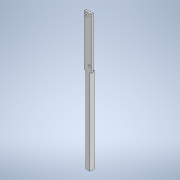
# Autodesk Inventor part: ArmV2
Saved by Autodesk Inventor 2021 (Build 250183000, 183)
## iProperties
Created: 2024-05-08
Part Number: ArmV2
Material: Generic
Document SubType Name: Modeling
Designer: brybr
Density: 1 g/cm^3
Appearance: Default
Author: brybr
Autodesk Inventor part; units mm, degrees
ref_plane "YZ Plane" through (0, 0, 0) normal (1, 0, 0) x (0, 1, 0)
ref_plane "XZ Plane" through (0, 0, 0) normal (0, 1, 0) x (-1, 0, 0)
ref_plane "XY Plane" through (0, 0, 0) normal (0, 0, 1) x (1, 0, 0)
sketch "Sketch1" plane through (0, 0, 0) normal (0, 0, 1) x (1, 0, 0)
  line L0 (-4, -30) -> (4, -30)
  line L1 (4, -30) -> (4, 30)
  line L2 (4, 30) -> (-4, 30)
  line L3 (-4, 30) -> (-4, -30)
  line L4 (-4, -30) -> (4, 30) construction
  line L5 (4, -30) -> (-4, 30) construction
  circle A0 centre (-2, 28) radius 1
  circle A1 centre (2, 28) radius 1
  circle A2 centre (-2, 25) radius 1
  circle A3 centre (2, -24) radius 1
  circle A4 centre (2, -23) radius 1
  point P0 (0, 0)
  point P1 (2.866, -23.5)
  point P2 (1.134, -23.5)
  dimension "d11" = 2
  dimension "d0" = 8
  dimension "d1" = 60
  dimension "d2" = 2
  dimension "d3" = 2
  dimension "d4" = 2
  dimension "d5" = 2
  dimension "d6" = 2
  dimension "d7" = 2
  dimension "d8" = 2
  dimension "d9" = 2
  dimension "d10" = 3
  dimension "d12" = 6
  dimension "d13" = 2
  dimension "d14" = 2
  constraints: 12 end point, 3 centre point, 2 midpoint, 2 parallel, 1 horizontal, 1 perpendicular, 6 other
  measures "d0" distance of L2.end L1.end
  measures "d1" distance of L1.end L0.end
  measures "d2" diameter of A0
  measures "d3" distance from line of L3 A0.centre
  measures "d4" distance from line of L2 A0.centre
  measures "d5" diameter of A1
  measures "d6" distance from line of L1 A1.centre
  measures "d7" distance from line of L2 A1.centre
  measures "d8" diameter of A2
  measures "d9" distance from line of L3 A2.centre
  measures "d10" distance of A2.centre A0.centre
  measures "d12" distance from line of L0 point (2, -24)
  measures "d13" distance from line of L1 point (2, -24)
  measures "d14" distance from line of L1 point (2, -23)
extrude "Extrusion1" add sketch "Sketch1" along normal blind 2
sketch "Sketch2" plane through (-4, -30, 0) normal (0, -1, 0) x (1, 0, 0)
  line L0 (1.6, 2) -> (6.4, 2)
  line L1 (6.4, 2) -> (6.4, -2.8)
  line L2 (6.4, -2.8) -> (1.6, -2.8)
  line L3 (1.6, -2.8) -> (1.6, 2)
  dimension "d21" = 4.8
  dimension "d22" = 4.8
  constraints: 8 end point, 2 parallel, 1 horizontal, 1 perpendicular
  measures "d21" distance of L1.end L2.end
  measures "d22" distance of L0.end L1.end
extrude "Extrusion2" add sketch "Sketch2" along normal blind 100
body "Solid1"
